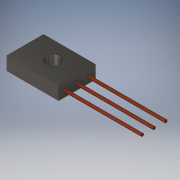
# Autodesk Inventor part: Transistor
Saved by Autodesk Inventor 2019 (Build 230136000, 136)
## iProperties
Created: 2020-05-07
Part Number: Transistor
Material: Copper, Alloy
Document SubType Name: Modeling
Designer: darkl
Density: 8.92 g/cm^3
Appearance: Copper - Satin
Author: darkl
Autodesk Inventor part; units mm, degrees
ref_plane "YZ Plane" through (0, 0, 0) normal (1, 0, 0) x (0, 1, 0)
ref_plane "XZ Plane" through (0, 0, 0) normal (0, 1, 0) x (-1, 0, 0)
ref_plane "XY Plane" through (0, 0, 0) normal (0, 0, 1) x (1, 0, 0)
sketch "Sketch1" plane through (0, 0, 0) normal (0, 1, 0) x (-1, 0, 0)
  line L0 (5.7156, 18.4944) -> (5.7156, 10.6944)
  line L1 (5.7156, 10.6944) -> (-5.2844, 10.6944)
  line L2 (-5.2844, 10.6944) -> (-5.2844, 18.4944)
  line L3 (-5.2844, 18.4944) -> (5.7156, 18.4944)
  point P0 (0, 0)
  dimension "d3" = 7.8
  dimension "d4" = 11
  dimension "d5" = 7.8
  dimension "d6" = 11
  constraints: 8 end point, 2 perpendicular, 1 vertical
  measures "d3" distance of L0.start L0.end
  measures "d4" distance of L0.end L1.end
  measures "d5" distance of L1.end L2.end
  measures "d6" distance of L2.end L0.start
extrude "Extrusion1" add sketch "Sketch1" along normal blind 2.8
sketch "Sketch2" plane through (5.2844, 0, 18.4944) normal (1, 0, 0) x (0, 0, -1)
  circle A0 centre (1.263, 1.3452) radius 0.3
  point P0 (18.4944, 0)
  dimension "d10" = 0.6
  constraints: 1 centre point
  measures "d10" diameter of A0
extrude "Extrusion2" add sketch "Sketch2" along normal blind 16.5
sketch "Sketch3" plane through (5.2844, 0, 18.4944) normal (1, 0, 0) x (0, 0, -1)
  circle A0 centre (1.263, 1.3452) radius 0.3 projected
  line L0 (1.263, 1.3452) -> (3.763, 1.3452)
  circle A1 centre (3.763, 1.3452) radius 0.3
  point P0 (18.4944, 0)
  dimension "d13" = 2.5
  dimension "d14" = 0.6
  constraints: 2 end point, 1 centre point, 1 coincident, 1 horizontal
  measures "d13" distance of L0.start L0.end
  measures "d14" diameter of A1
extrude "Extrusion3" add sketch "Sketch3" along normal blind 16.5 contours A1
sketch "Sketch4" plane through (5.2844, 0, 18.4944) normal (1, 0, 0) x (0, 0, -1)
  circle A0 centre (3.763, 1.3452) radius 0.3 projected
  line L0 (3.763, 1.3452) -> (6.263, 1.3452)
  circle A1 centre (6.263, 1.3452) radius 0.3
  point P0 (18.4944, 0)
  dimension "d17" = 2.5
  dimension "d18" = 0.6
  constraints: 2 end point, 1 centre point, 1 coincident, 1 horizontal
  measures "d17" distance of L0.start L0.end
  measures "d18" diameter of A1
extrude "Extrusion4" add sketch "Sketch4" along normal blind 16.5 contours A1
sketch "Sketch6" plane through (0, 2.8, 0) normal (0, 1, 0) x (1, 0, 0)
  circle A0 centre (0, -14.4314) radius 1.5 projected
  point P0 (0, 0)
  constraints: 1 coincident
hole "Hole1" at (0, 2.8, 14.4314) direction (0, -1, 0) diameter 3 end through all
body "Solid1"
